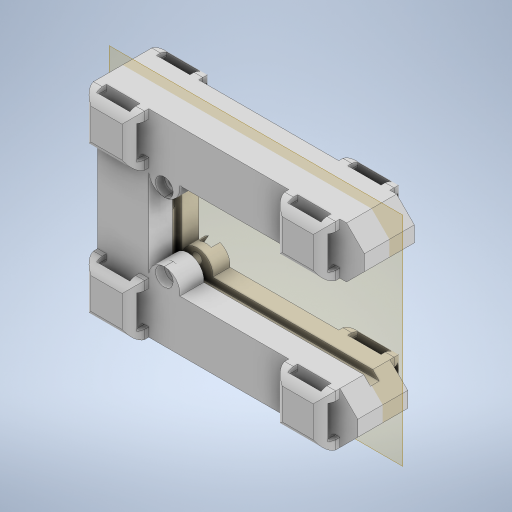
# Autodesk Inventor part: UCD Wire Bond V2 PCB Holder - U Shape
Saved by Autodesk Inventor 2024 (Build 280153000, 153)
## iProperties
Created: 2024-10-24
Part Number: UCD Wire Bond V2 PCB Holder - U Shape
Material: Generic
Document SubType Name: Modeling
Designer: Kemper Room 121
Density: 1 g/cm^3
Appearance: Default
Author: Kemper Room 121
Autodesk Inventor part; units mm, degrees
sketch "Sketch1" plane through (0, 0, 0) normal (0, 0, 1) x (1, 0, 0)
  line L0 (0, 0) -> (0, 10)
  line L1 (0, 10) -> (0, 34.5)
  line L2 (0, 34.5) -> (0, 44.5)
  line L3 (0, 44.5) -> (10, 44.5)
  line L4 (10, 44.5) -> (11.5, 44.5)
  line L5 (11.5, 44.5) -> (11.5, 11.5)
  line L6 (11.5, 11.5) -> (58.5, 11.5)
  line L7 (58.5, 0) -> (0, 0)
  line L8 (10, 44.5) -> (10, 10)
  line L9 (58.5, 11.5) -> (58.5, 10)
  line L10 (58.5, 10) -> (58.5, 0)
  line L11 (58.5, 0) -> (0, 0)
  line L12 (58.5, 10) -> (10, 10)
  line L13 (10, 44.5) -> (60, 44.5)
  line L14 (60, 44.5) -> (60, 34.5)
  line L15 (60, 34.5) -> (10, 34.5)
  line L16 (10, 34.5) -> (10, 44.5)
  line L17 (60, 34.5) -> (10, 34.5)
  line L18 (10, 34.5) -> (10, 33)
  line L19 (10, 33) -> (60, 33)
  line L20 (60, 33) -> (60, 34.5)
  point P0 (10.75, 44.5)
  point P1 (58.5, 10.75)
  point P2 (11.5, 33)
  dimension "d0" = 24.5
  dimension "d1" = 10
  dimension "d2" = 10
  dimension "d3" = 1.5
  dimension "d6" = 10
  dimension "d7" = 1.5
  dimension "d11" = 10
  dimension "d82" = 48.5
  dimension "d210" = 1.5
  dimension "d212" = 10
  constraints: 42 end point, 6 parallel, 6 perpendicular, 4 point on line, 3 horizontal, 2 midpoint, 2 vertical, 1 collinear
  measures "d0" distance of L0.end L1.end
  measures "d1" distance of L0.start L0.end
  measures "d2" distance of L2.end L3.end
  measures "d3" distance of L3.end L4.end
  measures "d6" distance of L9.end L7.start
  measures "d7" distance of L6.end L9.end
  measures "d11" distance of L1.end L2.end
  measures "d82" distance between parallel lines of L10 L8
  measures "d210" distance of L19.end L14.end
  measures "d212" distance between parallel lines of L13 L15
extrude "Extrusion1" add sketch "Sketch1" along normal blind 3.875
sketch "Sketch2" plane through (0, 0, 3.875) normal (0, 0, 1) x (1, 0, 0)
  line L0 (0, 0) -> (58.5, 0)
  line L1 (58.5, 0) -> (58.5, 11.5)
  line L2 (58.5, 11.5) -> (11.5, 11.5)
  line L3 (11.5, 11.5) -> (11.5, 33)
  line L4 (0, 44.5) -> (0, 0)
  line L5 (0, 0) -> (5.440208, 0)
  line L6 (10, 10) -> (10, 44.5)
  line L7 (10, 44.5) -> (0, 44.5)
  line L8 (0, 44.5) -> (0, 0)
  line L9 (58.5, 0) -> (58.5, 11.5)
  line L10 (0, 0) -> (58.5, 0)
  line L11 (58.5, 0) -> (58.5, 10)
  line L12 (58.5, 10) -> (10, 10)
  line L13 (0, -34.96781) -> (0, 0)
  line L14 (11.5, 33) -> (60, 33)
  line L15 (60, 33) -> (60, 44.5)
  line L16 (60, 44.5) -> (0, 44.5)
  line L17 (0, 44.5) -> (60, 44.5)
  line L18 (60, 44.5) -> (60, 34.5)
  line L19 (60, 34.5) -> (0, 34.5)
  line L20 (0, 34.5) -> (0, 44.5)
  point P0 (10, 34.5)
  dimension "d24" = 10
  dimension "d25" = 10
  dimension "d211" = 10
  constraints: 24 end point, 6 parallel, 3 horizontal, 3 perpendicular, 2 point on line
  measures "d24" distance of L6.end L4.start
  measures "d25" distance between parallel lines of L10 L12
  measures "d211" distance between parallel lines of L16 L19
extrude "Extrusion2" add sketch "Sketch2" along normal blind 2 contours L4 L19 L6 L12 L1 L0 | L4 L7 L6 L19 | L6 L16 L15 L19
sketch "Sketch5" plane through (0, 0, 5.875) normal (0, 0, 1) x (1, 0, 0)
  line L0 (0, 44.5) -> (0, 0) projected
  line L1 (0, 0) -> (58.5, 0) projected
  line L2 (58.5, 0) -> (58.5, 10) projected
  line L3 (10, 34.5) -> (10, 10) projected
  line L4 (10, 10) -> (58.5, 10) projected
  line L5 (58.5, 10) -> (58.5, 11.5) projected
  line L6 (58.5, 11.5) -> (11.5, 11.5) projected
  line L7 (11.5, 11.5) -> (11.5, 33) projected
  line L8 (0, 44.5) -> (11.5, 44.5)
  line L9 (16, 0) -> (0, 0)
  line L10 (0, 0) -> (0, 44.5)
  line L11 (0, 0) -> (58.5, 0)
  line L12 (58.5, 0) -> (58.5, 11.5)
  line L13 (58.5, 11.5) -> (11.5, 11.5)
  line L14 (0, -24) -> (0, 0)
  line L15 (11.5, 44.5) -> (11.5, 11.5)
  line L16 (60, 44.5) -> (0, 44.5) projected
  line L17 (60, 34.5) -> (60, 44.5) projected
  line L18 (60, 34.5) -> (10, 34.5) projected
  line L19 (11.5, 33) -> (60, 33) projected
  line L20 (60, 33) -> (60, 34.5) projected
  line L21 (58.5, 10) -> (10, 10) projected
  line L22 (10, 10) -> (10, 34.5) projected
  line L23 (10, 34.5) -> (60, 34.5) projected
  point P0 (11.5, 44.5)
  point P1 (10, 44.5)
  constraints: 17 end point, 4 parallel, 2 horizontal, 2 perpendicular, 1 point on line
extrude "Extrusion5" add sketch "Sketch5" along normal blind 5.375
sketch "Sketch6" plane through (0, 0, 0) normal (-1, 0, 0) x (0, 0, 1)
  line L0 (3.875, 34.5) -> (3.875, 10) projected
  line L1 (3.875, 10) -> (5.875, 10) projected
  line L2 (0, 44.5) -> (11.25, 44.5) projected
  line L3 (0, 44.5) -> (0, 0) projected
  line L4 (0, 0) -> (11.25, 0) projected
  line L5 (11.25, 44.5) -> (11.25, 0) projected
  circle A0 centre (5.625, 22.25) radius 2
  line L6 (3.875, 34.5) -> (5.875, 34.5) projected
  line L7 (5.875, 10) -> (5.875, 34.5) projected
  point P0 (5.875, 27.25)
  dimension "d52" = 4
  dimension "d53" = 11.25
  dimension "d54" = 5.625
  dimension "d213" = 44.5
  dimension "d214" = 22.25
  constraints: 1 centre point
  measures "d52" diameter of A0
  measures "d53" distance of L2.start L2.end
  measures "d54" distance from line of L3 A0.centre
  measures "d213" distance of L2.start L3.end
  measures "d214" distance from line of L4 A0.centre
extrude "Extrusion6" cut sketch "Sketch6" against normal blind 10 contours A0 L7 L0 | L0 A0 | A0 L7
sketch "Sketch7" plane through (0, 0, 0) normal (0, -1, 0) x (1, 0, 0)
  line L0 (10, 3.875) -> (58.5, 3.875) projected
  line L1 (10, 3.875) -> (10, 5.875) projected
  line L2 (58.5, 3.875) -> (58.5, 5.875) projected
  line L3 (0, 0) -> (0, 11.25) projected
  line L4 (0, 0) -> (58.5, 0) projected
  line L5 (58.5, 0) -> (58.5, 11.25) projected
  line L6 (0, 11.25) -> (58.5, 11.25) projected
  circle A0 centre (33.5, 5.625) radius 2
  circle A1 centre (22, 5.625) radius 2
  line L7 (58.5, 5.875) -> (10, 5.875) projected
  point P0 (58.5, 4.875)
  dimension "d60" = 4
  dimension "d61" = 4
  dimension "d62" = 11.25
  dimension "d63" = 5.625
  dimension "d64" = 5.625
  dimension "d77" = 12
  dimension "d78" = 23.5
  constraints: 2 centre point, 1 midpoint
  measures "d60" diameter of A0
  measures "d61" diameter of A1
  measures "d62" distance of L4.end L5.end
  measures "d63" distance from line of L4 A1.centre
  measures "d64" distance from line of L4 A0.centre
  measures "d77" distance from line of L1 A1.centre
  measures "d78" distance from line of L1 A0.centre
extrude "Extrusion7" [suppressed]
sketch "Sketch9" plane through (0, 0, 0) normal (0, 0, -1) x (-1, 0, 0)
  line L0 (0, 0) -> (-58.5, 0) projected
  line L1 (0, 44.5) -> (0, 0) projected
  line L2 (-11.5, 11.5) -> (-11.5, 33) projected
  line L3 (-58.5, 11.5) -> (-11.5, 11.5) projected
  line L4 (-58.5, 0) -> (-58.5, 11.5) projected
  circle A0 centre (-58.65, 11.5) radius 1.0625
  circle A1 centre (-11.5, 35.65) radius 1.0625
  line L5 (-60, 44.5) -> (0, 44.5) projected
  line L6 (-60, 33) -> (-60, 44.5) projected
  line L7 (-11.5, 33) -> (-60, 33) projected
  constraints: 2 centre point
extrude "Extrusion9" [suppressed]
sketch "Sketch10" plane through (0, 0, 11.25) normal (0, 0, 1) x (1, 0, 0)
  line L0 (10, 34.5) -> (10, 23.218246)
  line L1 (10, 10) -> (58.5, 10)
  line L2 (58.5, 10) -> (58.5, 11.5)
  line L3 (58.5, 11.5) -> (11.5, 11.5)
  line L4 (11.5, 11.5) -> (11.5, 33)
  line L5 (18.5, 13.5) -> (18.5, 23.072273)
  line L6 (18.5, 23.072273) -> (11.5, 23.072273)
  line L7 (11.5, 23.072273) -> (11.5, 13.5)
  arc A0 (11.5, 13.5) -> (18.5, 13.5) centre (15, 13.5) ccw
  circle A1 centre (15, 13.5) radius 1.125
  arc A2 (18.5, 11.5) -> (11.5, 11.5) centre (15, 11.96875) ccw
  line L8 (60, 34.5) -> (10, 34.5)
  line L9 (11.5, 33) -> (60, 33)
  line L10 (60, 33) -> (60, 34.5)
  line L11 (10, 23.218246) -> (10, 21.281754)
  line L12 (10, 21.281754) -> (10, 10)
  line L13 (14.078324, 15.5) -> (30.011363, 15.5)
  point P0 (0, 0)
  point P1 (15, 15.5)
  point P2 (11.56947, 12.806122)
  point P3 (18.43053, 12.806122)
  point P4 (17.872281, 11.5)
  point P5 (12.127719, 11.5)
  dimension "d90" = 2.25
  dimension "d215" = 3.5
  dimension "d216" = 5.5
  dimension "d217" = 5
  constraints: 8 end point, 5 point on circle, 4 point on line, 4 tangent, 3 centre point, 1 coincident, 1 horizontal, 1 parallel
  measures "d90" diameter of A1
  measures "d215" distance from line of L1 A0.centre
  measures "d216" distance between parallel lines of L1 L13
  measures "d217" distance from line of L12 A2.centre
extrude "Extrusion10" add sketch "Sketch10" against normal blind 11.25 contours A0 L3 | A0 A2 L3 | L3 L4 A2 A0 | A0 A2 L3 | A2 L4
ref_plane "Work Plane4" through (58.5, 22.25, 11.25) normal (0, 1, 0) x (1, 0, 0)
mirror "Mirror5" about plane through (58.5, 22.25, 11.25) normal (0, 1, 0) of "Extrusion10"
sketch "Sketch24" plane through (10, 34.5, 5.875) normal (1, 0, 0) x (0, 0, -1)
  line L0 (0, -1.5) -> (0, 0) projected
  line L1 (0, -1.5) -> (2, -1.5) projected
  line L2 (2, 0) -> (2, -1.5) projected
  line L3 (2, 0) -> (0, 0) projected
  line L4 (0, 0) -> (0, -1.5) projected
  line L5 (2, -1.5) -> (2, 0) projected
  line L6 (0, -1.5) -> (2, -1.5) projected
  line L7 (0, -24.5) -> (0, -23) projected
  line L8 (0, -24.5) -> (2, -24.5) projected
  line L9 (2, -23) -> (2, -24.5) projected
  line L10 (0, -23) -> (2, -23) projected
  line L11 (0, -23) -> (0, -24.5) projected
  line L12 (0, -23) -> (2, -23) projected
  line L13 (2, -24.5) -> (2, -23) projected
  line L14 (0, 0) -> (2, 0)
  line L15 (2, 0) -> (2, -24.5)
  line L16 (2, -24.5) -> (0, -24.5)
  line L17 (0, -24.5) -> (0, 0)
  point P0 (5.875, -34.5)
  constraints: 8 end point, 2 parallel, 1 horizontal, 1 perpendicular
extrude "Extrusion24" cut sketch "Sketch24" along normal through all
sketch "Sketch11" plane through (0, 0, 11.25) normal (0, 0, 1) x (1, 0, 0)
  arc A0 (18.5, 11.5) -> (11.5, 12.4375) centre (15, 11.96875) ccw
  circle A1 centre (15, 13.5) radius 1.125
  circle A2 centre (15, 13.5) radius 1.125
  line L0 (58.5, 11.5) -> (18.5, 11.5)
  line L1 (58.5, 0) -> (58.5, 11.5)
  line L2 (0, 0) -> (58.5, 0)
  line L3 (0, 44.5) -> (0, 0)
  line L4 (11.5, 12.4375) -> (11.5, 32.0625)
  line L5 (60, 44.5) -> (0, 44.5)
  line L6 (60, 33) -> (60, 44.5)
  line L7 (18.5, 33) -> (60, 33)
  arc A3 (11.5, 32.0625) -> (18.5, 33) centre (15, 32.53125) ccw
  constraints: 1 centre point, 1 coincident, 1 concentric
extrude "Extrusion11" [suppressed]
sketch "Sketch18" plane through (0, 0, 11.25) normal (0, 0, 1) x (1, 0, 0)
  line L0 (0, 11.5) -> (11.5, 11.5)
  line L1 (11.5, 11.5) -> (11.5, 0)
  line L2 (11.5, 0) -> (0, 0)
  line L3 (0, 0) -> (0, 11.5)
  line L4 (0, 0) -> (58.5, 0) projected
  line L5 (0, 44.5) -> (0, 0) projected
  line L6 (11.5, 12.4375) -> (11.5, 33) projected
  line L7 (58.5, 11.5) -> (18.5, 11.5) projected
  point P0 (11.5, 11.5)
  point P1 (11.5, 44.5)
  point P2 (5.75, 11.5)
  point P3 (18.627719, 11.5)
  dimension "d146" = 11.5
  dimension "d147" = 11.5
  dimension "d148" = 0
  dimension "d174" = 11.5
  dimension "d176" = 0
  dimension "d177" = 11.5
  constraints: 8 end point, 2 parallel, 1 horizontal, 1 midpoint, 1 perpendicular
  measures "d146" distance of L1.end L2.end
  measures "d147" distance of L0.end L1.end
  measures "d148" distance between parallel lines of L4 L2
  measures "d174" distance between parallel lines of L6 L5
  measures "d176" distance between parallel lines of L5 L3
  measures "d177" distance between parallel lines of L4 L7
extrude "Extrusion18" add sketch "Sketch18" along normal blind 5
pattern_linear "Rectangular Pattern2" count 2 spacing 33 along (0, 1, 0) of "Extrusion18"
pattern_linear "Rectangular Pattern3" count 2 spacing 43 along (1, 0, 0) of "Extrusion18", "Rectangular Pattern2"
ref_plane "Work Plane3" through (0, 0, 5.625) normal (0, 0, 1) x (1, 0, 0)
mirror "Mirror2" about plane through (0, 0, 5.625) normal (0, 0, 1) of "Extrusion18", "Rectangular Pattern2", "Rectangular Pattern3"
sketch "Sketch19" plane through (0, 0, 11.25) normal (0, -1, 0) x (-1, 0, 0)
  line L0 (-11.5, 0) -> (-43, 0)
  line L1 (-11.5, 0) -> (-11.5, -5)
  line L2 (0, -5) -> (-11.5, -5)
  line L3 (8.128246, -6.050437) -> (13.128246, -6.050437)
  line L4 (13.128246, -6.050437) -> (13.128246, -3.800437)
  line L5 (13.128246, -3.800437) -> (8.128246, -3.800437)
  line L6 (8.128246, -3.800437) -> (8.128246, -6.050437)
  line L7 (6.528996, -6.050437) -> (14.727497, -6.050437)
  line L8 (14.727497, -6.050437) -> (14.727497, -2.300437)
  line L9 (14.727497, -2.300437) -> (6.528996, -2.300437)
  line L10 (6.528996, -2.300437) -> (6.528996, -6.050437)
  line L11 (7.128246, -2.300437) -> (14.128246, -2.300437)
  line L12 (13.128246, -6.050437) -> (14.628246, -6.050437)
  line L13 (-11.5, 0) -> (-58.5, 0)
  line L14 (8.128246, -6.050437) -> (6.628246, -6.050437)
  arc A0 (7.128246, -2.300437) -> (6.628246, -6.050437) centre (12.684114, -4.949553) ccw
  arc A1 (14.628246, -6.050437) -> (14.128246, -2.300437) centre (8.572378, -4.949553) ccw
  line L15 (-11.5, 11.25) -> (-43, 11.25)
  line L16 (-58.5, 11.25) -> (-58.5, 0)
  line L17 (0, -5) -> (0, 16.25)
  line L18 (-54.5, 0) -> (-58.5, 0)
  line L19 (-54.5, 0) -> (-54.5, -5)
  line L20 (-43, -5) -> (-54.5, -5)
  line L21 (-43, 0) -> (-43, -5)
  line L22 (-43, 11.25) -> (-43, 16.25)
  line L23 (-43, 16.25) -> (-54.5, 16.25)
  line L24 (-54.5, 11.25) -> (-54.5, 16.25)
  line L25 (-54.5, 11.25) -> (-58.5, 11.25)
  line L26 (0, 16.25) -> (-11.5, 16.25)
  line L27 (-11.5, 11.25) -> (-11.5, 16.25)
  line L28 (22.439783, -2.25) -> (15.439783, -2.25)
  line L29 (22.439783, 0) -> (23.890831, 0)
  line L30 (15.439783, 0) -> (13.939783, 0)
  line L31 (15.439783, -2.25) -> (15.439783, 0)
  line L32 (22.439783, -2.25) -> (22.439783, 0)
  line L33 (-2, -2.25) -> (-9.5, -2.25)
  line L34 (-9.5, -2.25) -> (-9.5, 0)
  line L35 (-2, -2.25) -> (-2, 0)
  line L36 (-2.25, -3.75) -> (-9.25, -3.75)
  line L37 (-2, 0) -> (0, 0)
  line L38 (0, -5) -> (-11.5, -5)
  line L39 (0, 0) -> (-11.5, 0)
  line L40 (-9.5, 0) -> (-11.5, 0)
  line L41 (-11.5, 5.375) -> (-11.5, 0)
  arc A2 (-11.5, 0) -> (-9.25, -3.75) centre (-8.031556, -0.468934) ccw
  arc A3 (-2.25, -3.75) -> (0, 0) centre (-3.468444, -0.468934) ccw
  point P0 (0, 11.25)
  point P1 (10.628246, -2.300437)
  point P2 (10.628246, -3.800437)
  point P3 (10.628246, -2.300437)
  point P4 (-0.25, 0)
  point P5 (-13.09925, 0)
  point P6 (7.128246, -2.300437)
  point P7 (14.128246, -2.300437)
  point P8 (-11.59925, 0)
  point P9 (-19.59925, 0)
  point P10 (2.5, 3.75)
  point P11 (9.5, 3.75)
  point P12 (12, 1.918924)
  point P13 (6.628246, -6.050437)
  point P14 (10, 0)
  point P15 (6.528996, -4.949553)
  point P16 (2, 0)
  point P17 (-19.698501, 0)
  point P18 (14.727497, -4.949553)
  point P19 (-5.75, -5)
  point P20 (-5.75, -2.25)
  point P21 (-5.75, -5)
  point P22 (-5.75, -3.75)
  point P23 (-11.5, -0.937868)
  point P24 (0, -0.937868)
  dimension "d152" = 2.25
  dimension "d153" = 5
  dimension "d154" = 0
  dimension "d155" = 1.5
  dimension "d156" = 0
  dimension "d157" = 7
  dimension "d158" = 1.5
  dimension "d159" = 1.5
  dimension "d160" = 0
  dimension "d220" = 7
  dimension "d221" = 0
  dimension "d222" = 1.5
  dimension "d223" = 2.25
  dimension "d224" = 0
  dimension "d225" = 7
  dimension "d227" = 2
  dimension "d228" = 0
  dimension "d230" = 2.25
  dimension "d231" = 1.5
  dimension "d232" = 0
  dimension "d233" = 6.15512
  dimension "d234" = 0
  dimension "d235" = 2
  dimension "d236" = 3.5
  dimension "d237" = 3.5
  constraints: 44 end point, 8 point on circle, 7 midpoint, 6 horizontal, 4 centre point, 4 parallel, 3 perpendicular, 2 tangent, 1 collinear, 1 other
  measures "d152" distance of L3.end L4.end
  measures "d153" distance of L4.end L5.end
  measures "d154" horizontal distance of point (10.628, -2.3) point (10.628, -3.8)
  measures "d155" distance between parallel lines of L5 L9
  measures "d156" horizontal distance of point (10.628, -3.8) point (10.628, -2.3)
  measures "d157" distance of L11.start L11.end
  measures "d158" distance of L3.end L12.end
  measures "d159" distance of L3.start L14.end
  measures "d160" distance between parallel lines of L9 L11
  measures "d220" distance of L28.start L28.end
  measures "d221" distance from line of L30.start L31
  measures "d222" distance of L30.start L30.end
  measures "d223" distance of L28.end L31.end
  measures "d224" distance from line of L32 L29.start
  measures "d225" distance of L36.start L36.end
  measures "d227" distance of L35.end L37.end
  measures "d228" horizontal distance of point (-5.75, -5) point (-5.75, -2.25)
  measures "d230" distance of L33.end L34.end
  measures "d231" distance between parallel lines of L33 L36
  measures "d232" horizontal distance of point (-5.75, -5) point (-5.75, -3.75)
  measures "d233" radius of A0
  measures "d234" distance from line of L17 L37.end
  measures "d235" distance of L34.end L0.start
  measures "d236" radius of A2
  measures "d237" radius of A3
extrude "Extrusion19" cut sketch "Sketch19" against normal blind 12 contours A2 L36 A3 L17 L2 L1 | L39 L35 L33 L34
ref_plane "Work Plane1" through (1, 11.5, 11.25) normal (-1, 0, 0) x (0, 0, 1)
sketch "Sketch25" plane through (0, 11.5, 11.25) normal (-1, 0, 0) x (0, 0, 1)
  line L0 (0.937868, -11.5) -> (0.937868, 0)
  line L1 (0, 0) -> (0.937868, 0)
  line L2 (0, 21.5) -> (0, 0)
  line L3 (0, 21.5) -> (5, 21.5)
  line L4 (5, 33) -> (5, 21.5)
  line L5 (-16.25, 33) -> (5, 33)
  line L6 (-16.25, 33) -> (-16.25, 21.5)
  line L7 (-11.25, 21.5) -> (-16.25, 21.5)
  line L8 (-11.25, 21.5) -> (-11.25, 0)
  line L9 (-11.25, 0) -> (-16.25, 0)
  line L10 (-16.25, 0) -> (-16.25, -11.5)
  line L11 (0.937868, -11.5) -> (-16.25, -11.5)
  circle A0 centre (-5.625, 10.75) radius 2
  line L12 (2.25, -11.5) -> (2.25, 0)
  line L13 (0.937868, 0) -> (3.75, 0)
  line L14 (0.937868, -11.5) -> (0.937868, 0)
  line L15 (3.75, -11.5) -> (0.937868, -11.5)
  line L16 (3.75, -11.5) -> (3.75, 0)
  line L17 (0, -11.5) -> (0, 0)
  line L18 (0, -11.5) -> (5, -11.5)
  line L19 (5, 0) -> (5, -11.5)
  line L20 (0, 0) -> (5, 0)
  line L21 (0, -2) -> (2.25, -2)
  line L22 (2.25, -2) -> (2.25, -9.5)
  line L23 (2.25, -9.5) -> (0, -9.5)
  line L24 (0, -9.5) -> (0, -2)
  line L25 (3.75, -2.25) -> (3.75, -9.25)
  line L26 (0, -9.5) -> (0, -11.5)
  line L27 (0, -2) -> (0, 0)
  arc A1 (0, -11.5) -> (3.75, -9.25) centre (0.468934, -8.031556) ccw
  line L28 (0, 0) -> (0, 4)
  arc A2 (3.75, -2.25) -> (0, 0) centre (0.468934, -3.468444) ccw
  line L29 (0, -2) -> (2.25, -2)
  line L30 (0, -11.5) -> (0, 0)
  line L31 (2.25, -9.5) -> (2.25, -2)
  line L32 (0, -2) -> (0, -9.5)
  point P0 (-11.25, -11.5)
  point P1 (3.75, -5.75)
  point P2 (5, -5.75)
  point P3 (0, 0.9375)
  point P4 (3.75, -2.25)
  point P5 (3.75, -9.25)
  point P6 (0, -9.5)
  point P7 (2.25, -9.5)
  point P8 (2.25, -2)
  point P9 (0.937868, -2)
  dimension "d238" = 2
  dimension "d239" = 0
  dimension "d240" = 2
  dimension "d241" = 2.25
  dimension "d242" = 0
  dimension "d243" = 7
  dimension "d244" = 3.5
  dimension "d245" = 3.5
  dimension "d246" = 1.5
  constraints: 20 end point, 4 point on circle, 3 perpendicular, 2 centre point, 2 collinear, 2 midpoint, 2 parallel, 2 point on line, 1 horizontal, 1 vertical
  measures "d238" distance of L21.start L17.end
  measures "d239" distance from line of L18 L26.end
  measures "d240" distance of L23.end L26.end
  measures "d241" distance of L22.end L23.end
  measures "d242" vertical distance of point (3.75, -5.75) point (5, -5.75)
  measures "d243" distance of L25.start L25.end
  measures "d244" radius of A1
  measures "d245" radius of A2
  measures "d246" distance between parallel lines of L22 L25
extrude "Extrusion25" cut sketch "Sketch25" against normal blind 12 contours A1 L12 L15 | L23 L17 L21 L0 | L0 L21 L12 L23 | L12 A1 L16 L15 | L16 L20 L19 L18 | L13 L12 A2 | A2 L12 L13 L16
fillet "Fillet2" radius 1 4 edges at (9.5, 9.5, 12.375) (2, 2, 12.375) (2, 9.5, 12.375) (9.5, 2, 12.375)
pattern_linear "Rectangular Pattern5" count 2 spacing 33 along (0, 1, 0) count 2 spacing 43 along (1, 0, 0) of "Extrusion25", "Extrusion19", "Fillet2"
ref_plane "Work Plane2" through (0, 0, 5.625) normal (0, 0, 1) x (1, 0, 0)
mirror "Mirror6" about plane through (0, 0, 5.625) normal (0, 0, 1) of "Extrusion25", "Extrusion19", "Fillet2", "Rectangular Pattern5"
sketch "Sketch21" plane through (0, 0, 11.25) normal (0, 0, 1) x (1, 0, 0)
  circle A0 centre (15, 13.5) radius 2
  line L0 (60, 44.5) -> (54.5, 44.5)
  line L1 (11.5, 12.4375) -> (11.5, 32.0625)
  line L2 (60, 33) -> (60, 44.5)
  arc A1 (18.5, 11.5) -> (11.5, 12.4375) centre (15, 11.96875) ccw
  circle A2 centre (15, 13.5) radius 1.125
  arc A3 (11.5, 32.0625) -> (18.5, 33) centre (15, 32.53125) ccw
  line L3 (11.5, 44.5) -> (11.5, 42.5)
  line L4 (11.5, 33) -> (9.5, 33)
  line L5 (54.5, 33) -> (60, 33)
  line L6 (0, 33) -> (0, 11.5)
  line L7 (54.5, 44.5) -> (54.5, 42.5)
  line L8 (43, 33) -> (43, 35)
  line L9 (43, 44.5) -> (11.5, 44.5)
  line L10 (18.5, 33) -> (43, 33)
  line L11 (9.5, 11.5) -> (11.5, 11.5)
  line L12 (11.5, 11.5) -> (11.5, 9.5)
  line L13 (11.5, 0) -> (43, 0)
  line L14 (43, 0) -> (43, 2)
  line L15 (43, 11.5) -> (18.5, 11.5)
  line L16 (0, 11.5) -> (2, 11.5)
  line L17 (2, 0) -> (2, 1)
  line L18 (9.5, 0) -> (2, 0)
  line L19 (9.5, 0) -> (9.5, 1)
  line L20 (9.5, 10.5) -> (9.5, 11.5)
  line L21 (10.5, 9.5) -> (11.5, 9.5)
  line L22 (10.5, 2) -> (11.5, 2)
  line L23 (11.5, 2) -> (11.5, 0)
  line L24 (2, 10.5) -> (2, 11.5)
  line L25 (0, 9.5) -> (1, 9.5)
  line L26 (0, 2) -> (0, 9.5)
  line L27 (0, 2) -> (1, 2)
  arc A4 (9.5, 10.5) -> (10.5, 9.5) centre (10.5, 10.5) ccw
  arc A5 (1, 9.5) -> (2, 10.5) centre (1, 10.5) ccw
  arc A6 (2, 1) -> (1, 2) centre (1, 1) ccw
  arc A7 (10.5, 2) -> (9.5, 1) centre (10.5, 1) ccw
  line L28 (9.5, 33) -> (9.5, 34)
  arc A8 (10.5, 35) -> (9.5, 34) centre (10.5, 34) ccw
  line L29 (10.5, 35) -> (11.5, 35)
  line L30 (11.5, 35) -> (11.5, 33)
  line L31 (54.5, 35) -> (54.5, 33)
  line L32 (53.5, 42.5) -> (54.5, 42.5)
  arc A9 (52.5, 43.5) -> (53.5, 42.5) centre (53.5, 43.5) ccw
  line L33 (52.5, 43.5) -> (52.5, 44.5)
  line L34 (45, 44.5) -> (52.5, 44.5)
  line L35 (45, 43.5) -> (45, 44.5)
  arc A10 (44, 42.5) -> (45, 43.5) centre (44, 43.5) ccw
  line L36 (43, 42.5) -> (44, 42.5)
  line L37 (43, 42.5) -> (43, 44.5)
  line L38 (10.5, 42.5) -> (11.5, 42.5)
  arc A11 (9.5, 43.5) -> (10.5, 42.5) centre (10.5, 43.5) ccw
  line L39 (9.5, 43.5) -> (9.5, 44.5)
  line L40 (2, 44.5) -> (9.5, 44.5)
  line L41 (2, 43.5) -> (2, 44.5)
  arc A12 (1, 42.5) -> (2, 43.5) centre (1, 43.5) ccw
  line L42 (0, 42.5) -> (1, 42.5)
  line L43 (0, 35) -> (0, 42.5)
  line L44 (0, 35) -> (1, 35)
  arc A13 (2, 34) -> (1, 35) centre (1, 34) ccw
  line L45 (2, 33) -> (2, 34)
  line L46 (2, 33) -> (0, 33)
  line L47 (43, 2) -> (44, 2)
  arc A14 (45, 1) -> (44, 2) centre (44, 1) ccw
  line L48 (45, 0) -> (45, 1)
  line L49 (52.5, 0) -> (45, 0)
  line L50 (52.5, 0) -> (52.5, 1)
  arc A15 (53.5, 2) -> (52.5, 1) centre (53.5, 1) ccw
  line L51 (53.5, 2) -> (54.5, 2)
  line L52 (54.5, 2) -> (54.5, 0)
  line L53 (54.5, 0) -> (58.5, 0)
  line L54 (58.5, 0) -> (58.5, 11.5)
  line L55 (58.5, 11.5) -> (54.5, 11.5)
  line L56 (54.5, 11.5) -> (54.5, 9.5)
  line L57 (53.5, 9.5) -> (54.5, 9.5)
  arc A16 (52.5, 10.5) -> (53.5, 9.5) centre (53.5, 10.5) ccw
  line L58 (52.5, 10.5) -> (52.5, 11.5)
  line L59 (45, 11.5) -> (52.5, 11.5)
  line L60 (45, 10.5) -> (45, 11.5)
  arc A17 (44, 9.5) -> (45, 10.5) centre (44, 10.5) ccw
  line L61 (43, 9.5) -> (44, 9.5)
  line L62 (43, 9.5) -> (43, 11.5)
  line L63 (43, 35) -> (44, 35)
  arc A18 (45, 34) -> (44, 35) centre (44, 34) ccw
  line L64 (45, 33) -> (45, 34)
  line L65 (52.5, 33) -> (45, 33)
  line L66 (52.5, 33) -> (52.5, 34)
  arc A19 (53.5, 35) -> (52.5, 34) centre (53.5, 34) ccw
  line L67 (53.5, 35) -> (54.5, 35)
  circle A20 centre (15, 31) radius 1.125
  circle A21 centre (15, 31) radius 2
  point P0 (0, 0)
  dimension "d193" = 4
  dimension "d256" = 0
  dimension "d257" = 4
  constraints: 2 centre point, 1 coincident
  measures "d193" diameter of A0
  measures "d256" distance of A2.centre A0.centre
  measures "d257" diameter of A21
extrude "Extrusion21" cut sketch "Sketch21" against normal blind 2 contours A0 | A21 | A2
chamfer "Chamfer1" distance 4 angle 45 4 edges at (60, 33, 8.5625) (60, 44.5, 5.625) (58.5, 11.5, 8.5625) (58.5, 0, 5.625)
sketch "Sketch26" plane through (0, 0, 0) normal (0, 0, -1) x (-1, 0, 0)
  line L0 (-54.5, 0) -> (-58.5, 4)
  line L1 (-54.5, 0) -> (-54.5, 2)
  line L2 (-53.5, 2) -> (-54.5, 2)
  arc A0 (-52.5, 1) -> (-53.5, 2) centre (-53.5, 1) ccw
  line L3 (-52.5, 0) -> (-52.5, 1)
  line L4 (-45, 0) -> (-52.5, 0)
  line L5 (-45, 0) -> (-45, 1)
  arc A1 (-44, 2) -> (-45, 1) centre (-44, 1) ccw
  line L6 (-43, 2) -> (-44, 2)
  line L7 (-43, 2) -> (-43, 0)
  line L8 (-11.5, 0) -> (-43, 0)
  line L9 (-11.5, 0) -> (-11.5, 2)
  line L10 (-10.5, 2) -> (-11.5, 2)
  arc A2 (-9.5, 1) -> (-10.5, 2) centre (-10.5, 1) ccw
  line L11 (-9.5, 0) -> (-9.5, 1)
  line L12 (-2, 0) -> (-9.5, 0)
  line L13 (-2, 0) -> (-2, 1)
  arc A3 (-1, 2) -> (-2, 1) centre (-1, 1) ccw
  line L14 (0, 2) -> (-1, 2)
  line L15 (0, 9.5) -> (0, 2)
  line L16 (0, 9.5) -> (-1, 9.5)
  arc A4 (-2, 10.5) -> (-1, 9.5) centre (-1, 10.5) ccw
  line L17 (-2, 10.5) -> (-2, 11.5)
  line L18 (-2, 11.5) -> (0, 11.5)
  line L19 (0, 33) -> (0, 11.5)
  line L20 (0, 33) -> (-2, 33)
  line L21 (-2, 33) -> (-2, 34)
  arc A5 (-1, 35) -> (-2, 34) centre (-1, 34) ccw
  line L22 (0, 35) -> (-1, 35)
  line L23 (0, 42.5) -> (0, 35)
  line L24 (0, 42.5) -> (-1, 42.5)
  arc A6 (-2, 43.5) -> (-1, 42.5) centre (-1, 43.5) ccw
  line L25 (-2, 43.5) -> (-2, 44.5)
  line L26 (-9.5, 44.5) -> (-2, 44.5)
  line L27 (-9.5, 43.5) -> (-9.5, 44.5)
  arc A7 (-10.5, 42.5) -> (-9.5, 43.5) centre (-10.5, 43.5) ccw
  line L28 (-10.5, 42.5) -> (-11.5, 42.5)
  line L29 (-11.5, 42.5) -> (-11.5, 44.5)
  line L30 (-43, 44.5) -> (-11.5, 44.5)
  line L31 (-43, 44.5) -> (-43, 42.5)
  line L32 (-43, 42.5) -> (-44, 42.5)
  arc A8 (-45, 43.5) -> (-44, 42.5) centre (-44, 43.5) ccw
  line L33 (-45, 43.5) -> (-45, 44.5)
  line L34 (-52.5, 44.5) -> (-45, 44.5)
  line L35 (-52.5, 43.5) -> (-52.5, 44.5)
  arc A9 (-53.5, 42.5) -> (-52.5, 43.5) centre (-53.5, 43.5) ccw
  line L36 (-53.5, 42.5) -> (-54.5, 42.5)
  line L37 (-54.5, 42.5) -> (-54.5, 44.5)
  line L38 (-56, 44.5) -> (-54.5, 44.5)
  line L39 (-60, 40.5) -> (-56, 44.5)
  line L40 (-60, 37) -> (-60, 40.5)
  line L41 (-56, 33) -> (-60, 37)
  line L42 (-54.5, 33) -> (-56, 33)
  line L43 (-54.5, 33) -> (-54.5, 35)
  line L44 (-53.5, 35) -> (-54.5, 35)
  arc A10 (-52.5, 34) -> (-53.5, 35) centre (-53.5, 34) ccw
  line L45 (-52.5, 33) -> (-52.5, 34)
  line L46 (-45, 33) -> (-52.5, 33)
  line L47 (-45, 33) -> (-45, 34)
  arc A11 (-44, 35) -> (-45, 34) centre (-44, 34) ccw
  line L48 (-43, 35) -> (-44, 35)
  line L49 (-43, 35) -> (-43, 33)
  line L50 (-18.5, 33) -> (-43, 33)
  arc A12 (-18.5, 33) -> (-11.5, 32.0625) centre (-15, 32.53125) ccw
  line L51 (-11.5, 12.4375) -> (-11.5, 32.0625)
  arc A13 (-11.5, 12.4375) -> (-18.5, 11.5) centre (-15, 11.96875) ccw
  line L52 (-43, 11.5) -> (-18.5, 11.5)
  line L53 (-43, 11.5) -> (-43, 9.5)
  line L54 (-43, 9.5) -> (-44, 9.5)
  arc A14 (-45, 10.5) -> (-44, 9.5) centre (-44, 10.5) ccw
  line L55 (-45, 10.5) -> (-45, 11.5)
  line L56 (-52.5, 11.5) -> (-45, 11.5)
  line L57 (-52.5, 10.5) -> (-52.5, 11.5)
  arc A15 (-53.5, 9.5) -> (-52.5, 10.5) centre (-53.5, 10.5) ccw
  line L58 (-53.5, 9.5) -> (-54.5, 9.5)
  line L59 (-54.5, 9.5) -> (-54.5, 11.5)
  line L60 (-58.5, 7.5) -> (-54.5, 11.5)
  line L61 (-58.5, 4) -> (-58.5, 7.5)
  line L62 (-9.5, 33) -> (-11.5, 33)
  line L63 (-11.5, 33) -> (-11.5, 35)
  line L64 (-10.5, 35) -> (-11.5, 35)
  arc A16 (-9.5, 34) -> (-10.5, 35) centre (-10.5, 34) ccw
  line L65 (-9.5, 33) -> (-9.5, 34)
  circle A17 centre (-15, 13.5) radius 1.125
  circle A18 centre (-15, 31) radius 1.125
  line L66 (-11.5, 9.5) -> (-11.5, 11.5)
  line L67 (-11.5, 11.5) -> (-9.5, 11.5)
  line L68 (-9.5, 10.5) -> (-9.5, 11.5)
  arc A19 (-10.5, 9.5) -> (-9.5, 10.5) centre (-10.5, 10.5) ccw
  line L69 (-10.5, 9.5) -> (-11.5, 9.5)
  line L70 (-17.309401, 13.5) -> (-16.154701, 15.5)
  line L71 (-16.154701, 15.5) -> (-13.845299, 15.5)
  line L72 (-13.845299, 15.5) -> (-12.690599, 13.5)
  line L73 (-12.690599, 13.5) -> (-13.845299, 11.5)
  line L74 (-13.845299, 11.5) -> (-16.154701, 11.5)
  line L75 (-16.154701, 11.5) -> (-17.309401, 13.5)
  line L76 (-17.309401, 31) -> (-16.154701, 33)
  line L77 (-16.154701, 33) -> (-13.845299, 33)
  line L78 (-13.845299, 33) -> (-12.690599, 31)
  line L79 (-12.690599, 31) -> (-13.845299, 29)
  line L80 (-13.845299, 29) -> (-16.154701, 29)
  line L81 (-16.154701, 29) -> (-17.309401, 31)
  point P0 (0, 0)
  point P1 (-15, 29)
  dimension "d262" = 4
  dimension "d263" = 4
  dimension "d264" = 90
  dimension "d265" = 90
  constraints: 24 end point, 2 coincident, 26 other
  measures "d262" distance between parallel lines of L74 L71
  measures "d263" distance between parallel lines of L80 L77
  measures "d264" angle of L51 L77
  measures "d265" angle of L51 L71
extrude "Extrusion26" cut sketch "Sketch26" against normal blind 2 contours L70 L71 A13 | A13 L72 L73 L74 L75 L70 | L71 L72 A13 | L79 L80 A12 | A12 L81 L76 L77 L78 L79 | L80 L81 A12 | A17 | A18
equation "\"d1\" = Clamp_Bracket_W"
equation "\"d2\" = Clamp_Bracket_W"
equation "\"d3\" = Trim_Mount_W"
equation "\"d6\" = d1"
equation "\"d7\" = d3"
equation "\"d82\" = PCB_L_Offset + PCB_L + Trim_Mount_W"
equation "\"d22\" = Mount_W_Back"
equation "\"d24\" = Clamp_Bracket_W"
equation "\"d25\" = Clamp_Bracket_W"
equation "\"d52\" = d51"
equation "\"d54\" = 0.5 * d53"
equation "\"d58\" = Clamp_Bracket_W"
equation "\"d60\" = d51"
equation "\"d61\" = d51"
equation "\"d63\" = 0.5 * d62"
equation "\"d64\" = 0.5 * d62"
equation "\"d77\" = 0.5 * PCB_W + PCB_W_Offset"
equation "\"d78\" = 0.5 * PCB_L"
equation "\"d67\" = Clamp_Bracket_W"
equation "\"Clamp_Bracket_W\" = 10"
equation "\"Trim_Mount_W\" = 1.5"
equation "\"PCB_L_Offset\" = 0"
equation "\"PCB_L\" = 47"
equation "\"Mount_W_Back\" = 3.875"
equation "\"d51\" = 4"
equation "\"PCB_W\" = 24"
equation "\"PCB_W_Offset\" = 0"
body "Solid1"
